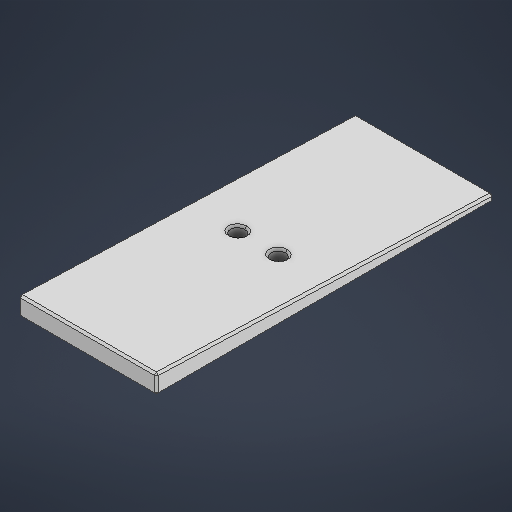
# Autodesk Inventor part: Game-Piece-Funnel-Pusher-Plate
Saved by Autodesk Inventor 2025 (Build 290162010, 162A)
## iProperties
Created: 2025-11-05
Part Number: Game-Piece-Funnel-Pusher-Plate
Material: Generic
Document SubType Name: Modeling
Designer: FizzyApple12
Density: 1 g/cm^3
Appearance: Default
Author: FizzyApple12
Autodesk Inventor part; units mm, degrees
ref_plane "YZ Plane" through (0, 0, 0) normal (1, 0, 0) x (0, 1, 0)
ref_plane "XZ Plane" through (0, 0, 0) normal (0, 1, 0) x (-1, 0, 0)
sketch "Sketch1" plane through (0, 0, 0) normal (0, 1, 0) x (-1, 0, 0)
  line L0 (0, 0) -> (-34, 0)
  line L1 (-34, 0) -> (-34, -83)
  line L2 (-34, -83) -> (0, -83)
  line L3 (0, -83) -> (0, 0)
  line L4 (-10, -40) -> (-24, -40)
  line L5 (-24, -40) -> (-24, -44)
  line L6 (-24, -44) -> (-10, -44)
  line L7 (-10, -44) -> (-10, -40)
  line L8 (-17, 0) -> (-17, -40) construction
  line L9 (-10, -44) -> (-14, -40) construction
  line L10 (-24, -44) -> (-20, -40) construction
  point P0 (-22, -42)
  point P1 (-12, -42)
  dimension "d0" = 34
  dimension "d1" = 83
  dimension "d2" = 14
  dimension "d3" = 4
  dimension "d4" = 43
  dimension "d12" = 45
  constraints: 22 end point, 4 midpoint, 4 parallel, 4 perpendicular, 2 horizontal, 2 point on line
  measures "d0" distance of L2.end L1.end
  measures "d1" distance of L0.end L1.end
  measures "d2" distance of L6.end L5.end
  measures "d3" distance of L5.end L4.end
  measures "d4" distance between parallel lines of L2 L4
  measures "d12" angle of L5 L10
extrude "Extrusion1" add sketch "Sketch1" along normal blind 1.8 contours L3 L2 L1 L0 | L7 L6 L5 L4
extrude "Extrusion2" add sketch "Sketch1" against normal blind 3.4 contours L7 L6 L5 L4
ref_plane "Work Plane1" through (34, 1.8, -83) normal (0, 0.9993908, -0.0348995) x (-1, 0, 0)
extrude "Extrusion3" add sketch "Sketch1" along normal up to surface contours L3 L2 L1 L0 | L7 L6 L5 L4 surface through (34, 1.8, -83) normal (0, 0.9993908, -0.0348995)
sketch "Sketch2" plane through (0, -3.4, 0) normal (0, -1, 0) x (1, 0, 0)
  point P0 (0, 0)
  point P1 (22, -42)
  point P2 (12, -42)
hole "Hole1" at (22, -3.4, -42) at (12, -3.4, -42) direction (0, 1, 0) diameter 3.5 depth 8
fillet "Fillet1" radius 2 4 edges at (24, -1.7, -40) (24, -1.7, -44) (10, -1.7, -40) (10, -1.7, -44)
chamfer "Chamfer1" distance 0.5 angle 45 22 edges at (17, 4.6984, 0) (0, 3.2492, -41.5) (34, 3.2492, -41.5) (34, 0, -41.5) (34, 2.3492, 0) (17, 0, 0) (0, 0, -41.5) (17, 0, -83) (17, 1.8, -83) (0, 0.9, -83) (34, 0.9, -83) (0, 2.3492, 0) (22, 3.2929, -40.25) (12, 3.2929, -40.25) (10.5858, 0, -40.5858) (10, 0, -42) (10.5858, 0, -43.4142) (17, 0, -44) (23.4142, 0, -40.5858) (24, 0, -42) (23.4142, 0, -43.4142) (17, 0, -40)
body "Solid1"
